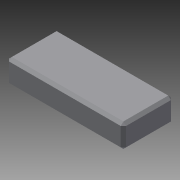
# Autodesk Inventor part: Battery_3.7V
Saved by Autodesk Inventor 2015 (Build 190159000, 159)
## iProperties
Created: 2015-02-13
Part Number: Battery_3.7V
Material: Generic
Document SubType Name: Modeling
Designer: Judson
Density: 1 g/cm^3
Appearance: Default
Author: Judson
Autodesk Inventor part; units mm, degrees
ref_plane "YZ Plane" through (0, 0, 0) normal (1, 0, 0) x (0, 1, 0)
ref_plane "XZ Plane" through (0, 0, 0) normal (0, 1, 0) x (-1, 0, 0)
ref_plane "XY Plane" through (0, 0, 0) normal (0, 0, 1) x (1, 0, 0)
sketch "Sketch1" plane through (0, 0, 0) normal (0, 1, 0) x (-1, 0, 0)
  line L0 (25, 4.9474) -> (-3, 4.9474)
  line L1 (-3, 4.9474) -> (-3, -7.0526)
  line L2 (-3, -7.0526) -> (25, -7.0526)
  line L3 (25, -7.0526) -> (25, 4.9474)
  point P0 (0, 0)
  dimension "d0" = 12
  dimension "d1" = 28
  constraints: 8 end point, 2 parallel, 1 horizontal, 1 perpendicular
  measures "d0" distance of L0.end L1.end
  measures "d1" distance of L1.end L2.end
extrude "Extrusion1" add sketch "Sketch1" along normal blind 5.7
chamfer "Chamfer1" distance 0.635 angle 45 12 edges at (-11, 5.7, 4.9474) (-11, 5.7, -7.0526) (3, 5.7, -1.0526) (-11, 0, 4.9474) (3, 0, -1.0526) (3, 2.85, -7.0526) (3, 2.85, 4.9474) (-11, 0, -7.0526) (-25, 2.85, -7.0526) (-25, 0, -1.0526) (-25, 5.7, -1.0526) (-25, 2.85, 4.9474)
body "Solid1"
